Back Plate (Autodesk Fusion 360 design; units mm, degrees)
part number: Back Plate
Autodesk Fusion 360 part; units mm, degrees
sketch "Sketch1" plane through (0, 0, 0) normal (0, 0, 1) x (1, 0, 0)
  line L0 (0, 0) -> (-140, 0)
  line L1 (-140, 0) -> (-140, 52)
  line L2 (-140, 52) -> (0, 52)
  line L3 (0, 52) -> (0, 0)
  line L4 (0, -5) -> (-140, -5)
  line L5 (-145, 0) -> (-145, 52)
  line L6 (-140, 57) -> (0, 57)
  line L7 (5, 52) -> (5, 0)
  line L8 (-63, 19) -> (-77, 19)
  line L9 (-58, 28) -> (-58, 24)
  arc A0 (-77, 33) -> (-82, 28) centre (-77, 28) ccw
  arc A1 (-82, 24) -> (-77, 19) centre (-77, 24) ccw
  arc A2 (-63, 19) -> (-58, 24) centre (-63, 24) ccw
  line L10 (-82, 24) -> (-82, 28)
  line L11 (-77, 33) -> (-63, 33)
  arc A3 (-58, 28) -> (-63, 33) centre (-63, 28) ccw
  arc A4 (0, -5) -> (5, 0) centre (0, 0) ccw
  arc A5 (5, 52) -> (0, 57) centre (0, 52) ccw
  arc A6 (-140, 57) -> (-145, 52) centre (-140, 52) ccw
  arc A7 (-145, 0) -> (-140, -5) centre (-140, 0) ccw
  point P0 (-82, 19)
  point P1 (-82, 33)
  point P2 (-58, 33)
  dimension "d1" = 140
  dimension "d2" = 52
  dimension "d4" = 24
  dimension "d5" = 14
  dimension "d7" = 5
  dimension "d8" = 5
  dimension "d9" = 19
  dimension "d10" = 58
  dimension "d11" = 5
  constraint horizontal L0
  constraint vertical L1
  constraint horizontal L2
  constraint vertical L3
  constraint coincident L0.start L3.end
  constraint horizontal L11
  constraint vertical L9
  constraint horizontal L8
  constraint vertical L10
  constraint coincident P2 L11
  constraint coincident P2 L9
  constraint tangent L11 A3
  constraint tangent L9 A3
  constraint tangent L9 A2
  constraint tangent L8 A2
  constraint equal A2 A3
  constraint coincident P0 L8
  constraint coincident P0 L10
  constraint tangent L8 A1
  constraint tangent A1 L10
  constraint equal A1 A3
  constraint coincident P1 L11
  constraint coincident P1 L10
  constraint tangent A0 L11
  constraint tangent A0 L10
  constraint parallel L0 L4
  constraint parallel L1 L5
  constraint parallel L2 L6
  constraint parallel L3 L7
  constraint tangent L4 A4
  constraint tangent L7 A4
  constraint tangent L6 A5
  constraint tangent L7 A5
  constraint equal A4 A5
  constraint tangent L5 A6
  constraint tangent L6 A6
  constraint equal A4 A6
  constraint tangent L4 A7
  constraint tangent L5 A7
  constraint equal A4 A7
  measures "d1" distance of L0.start L0.end
  measures "d2" distance of L0.start L2.end
  measures "d4" distance of P1 P2
  measures "d5" distance of P0 P1
  measures "d7" radius of A3
  measures "d8" radius of A0
  measures "d9" distance of L2 L11
  measures "d10" distance of L3 L9
  measures "d11" radius of A4
extrude "Extrude1" add sketch "Sketch1" along normal blind 10 contours L0 L1 L2 L3
fillet "Fillet1" radius 5 8 edges at (-82, 26, 0) (-80.5355, 31.5355, 0) (-70, 33, 0) (-59.4645, 31.5355, 0) (-58, 26, 0) (-59.4645, 20.4645, 0) (-70, 19, 0) (-80.5355, 20.4645, 0)
extrude "Extrude2" add sketch "Sketch1" along normal blind 2 contours L4 L5 L6 L7 A4 A5 A6 A7
